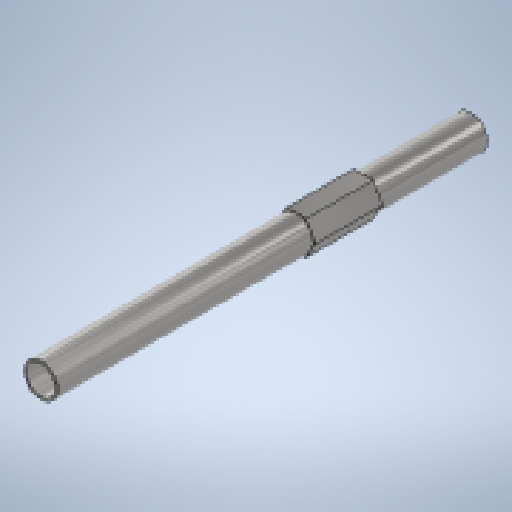
# Autodesk Inventor part: Shaft
Saved by Autodesk Inventor 2023.2 (Build 272271000, 271)
## iProperties
Created: 2024-03-17
Part Number: Shaft
Material: Stainless Steel
Document SubType Name: Modeling
Designer: Nathan Cai
Mass: 11.5588 g
Surface Area: 47.5925 cm^2
Volume: 1.44485 cm^3
Density: 8 g/cm^3
Appearance: Semi-Polished
Author: Nathan Cai
Autodesk Inventor part; units mm, degrees
ref_plane "YZ Plane" through (0, 0, 0) normal (1, 0, 0) x (0, 1, 0)
ref_plane "XZ Plane" through (0, 0, 0) normal (0, 1, 0) x (-1, 0, 0)
sketch "Sketch1" plane through (0, 0, 0) normal (0, 0, 1) x (1, 0, 0)
  line L0 (2.2914, 3.9688) -> (4.5827, 0)
  line L1 (4.5827, 0) -> (2.2914, -3.9687)
  line L2 (2.2914, -3.9687) -> (-2.2914, -3.9687)
  line L3 (-2.2914, -3.9687) -> (-4.5827, 0)
  line L4 (-4.5827, 0) -> (-2.2914, 3.9688)
  line L5 (-2.2914, 3.9688) -> (2.2914, 3.9688)
  circle A0 centre (0, 0) radius 3.375
  dimension "d0" = 7.9375
  dimension "d1" = 6.75
  constraints: 12 end point, 2 coincident, 1 centre point, 1 horizontal, 13 other
  measures "d0" distance between parallel lines of L2 L5
  measures "d1" diameter of A0
extrude "Extrusion1" add sketch "Sketch1" along normal blind 101.6
sketch "Sketch2" plane through (0, 0, 0) normal (0, 0, -1) x (-1, 0, 0)
  circle A0 centre (0, 0) radius 3.925
  line L0 (2.2914, 3.9688) -> (4.5827, 0) projected
  line L1 (-2.2914, 3.9688) -> (2.2914, 3.9688) projected
  line L2 (-4.5827, 0) -> (-2.2914, 3.9688) projected
  line L3 (-2.2914, -3.9687) -> (-4.5827, 0) projected
  line L4 (2.2914, -3.9687) -> (-2.2914, -3.9687) projected
  line L5 (4.5827, 0) -> (2.2914, -3.9687) projected
  circle A1 centre (0, 0) radius 3.375 projected
  dimension "d4" = 7.85
  constraints: 1 centre point, 1 coincident
  measures "d4" diameter of A0
extrude "Extrusion2" cut sketch "Sketch2" against normal blind 25.4 contours L0 L5 L4 L3 L2 L1
ref_plane "Work Plane1" through (0, 0, 41.275) normal (0, 0, -1) x (-1, 0, 0)
sketch "Sketch3" plane through (0, 0, 41.275) normal (0, 0, -1) x (-1, 0, 0)
  line L0 (-4.5827, 0) -> (-2.2914, 3.9688) projected
  line L1 (-2.2914, -3.9687) -> (-4.5827, 0) projected
  line L2 (2.2914, -3.9687) -> (-2.2914, -3.9687) projected
  line L3 (4.5827, 0) -> (2.2914, -3.9687) projected
  line L4 (2.2914, 3.9688) -> (4.5827, 0) projected
  line L5 (-2.2914, 3.9688) -> (2.2914, 3.9688) projected
  circle A0 centre (0, 0) radius 3.925 projected
  circle A1 centre (0, 0) radius 3.9688
  point P0 (-3.437, -1.9844)
  point P1 (-3.437, 1.9844)
  point P2 (0, 3.9688)
  point P3 (3.437, 1.9844)
  point P4 (3.437, -1.9844)
  point P5 (0, -3.9688)
  constraints: 1 centre point, 1 coincident, 1 tangent
extrude "Extrusion3" cut sketch "Sketch3" against normal through all contours L0 A1 L1 | L0 L5 A1 | A1 L2 L1 | L5 L4 A1 | A1 L3 L2 | L4 L3 A1
body "Solid1"
